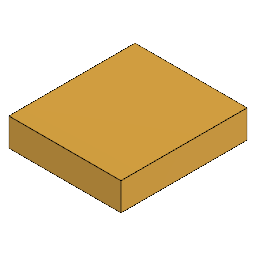
vr_trackers_case (Autodesk Fusion 360 archive; units mm, degrees)
design "ASR00007 battery"
part number: 2026-03-05-17-50-04-894
Autodesk Fusion 360 part; units mm, degrees
sketch "Sketch1" plane through (0, 0, 0) normal (0, 0, 1) x (1, 0, 0)
  line L0 (0, 0) -> (24, 0)
  line L1 (24, 0) -> (24, 27)
  line L2 (24, 27) -> (0, 27)
  line L3 (0, 27) -> (0, 0)
  dimension "d1" = 27
  dimension "d2" = 24
  constraint horizontal L0
  constraint vertical L1
  constraint horizontal L2
  constraint vertical L3
  constraint coincident L0.start L3.end
  measures "d1" distance of L0.start L2.end
  measures "d2" distance of L0.start L0.end
extrude "Extrude1" add sketch "Sketch1" along normal blind 6
